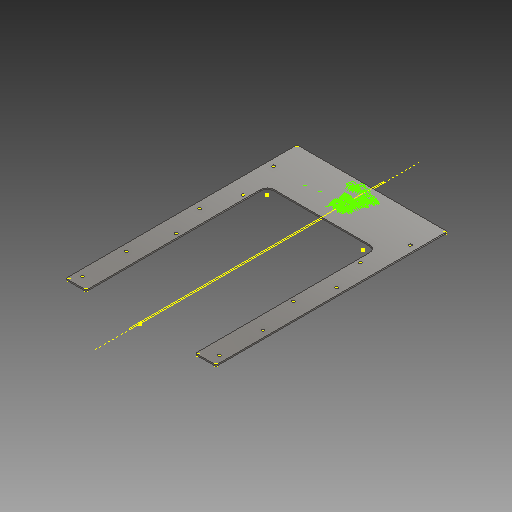
# Autodesk Inventor part: Front
Saved by Autodesk Inventor 2018 (Build 220112000, 112)
## iProperties
Created: 2017-10-08
Part Number: Front
Material: Edelstahl
Document SubType Name: Blech
Designer: jro
Density: 8 g/cm^3
Sheet Metal Rule: Standard_mm
Appearance: Halbpoliert
Mass: 436.49 g
Surface Area: 580.02 cm^2
Volume: 54.5612 cm^3
Flat Pattern Width: 22.4 cm
Flat Pattern Length: 34.5 cm
Flat Pattern Area: 772.799 cm^2
Sheet Metal Width: 224,000 mm
Sheet Metal Length: 345,000 mm
Sheet Metal Area: 77279,943 mm^2
Author: jro
Autodesk Inventor part; units mm, degrees
(part 1 of 2)
ref_plane "YZ Plane" through (0, 0, 0) normal (1, 0, 0) x (0, 1, 0)
ref_plane "XZ Plane" through (0, 0, 0) normal (0, 1, 0) x (-1, 0, 0)
ref_plane "XY Plane" through (0, 0, 0) normal (0, 0, 1) x (1, 0, 0)
sketch "Skizze1" plane through (0, 0, 0) normal (0, 0, 1) x (1, 0, 0)
  line L0 (106.9629, 2) -> (-106.9629, 2)
  line L1 (0, -19.6018) -> (0, 5.6106)
  line L2 (0, 2) -> (81.5, 2)
  line L3 (0, 2) -> (-81.5, 2)
  line L4 (-81.5, 2) -> (-81.5, 262)
  line L5 (81.5, 2) -> (81.5, 262)
  line L6 (71.5, 272) -> (-71.5, 272)
  arc A0 (81.5, 262) -> (71.5, 272) centre (71.5, 262) ccw
  arc A1 (-71.5, 272) -> (-81.5, 262) centre (-71.5, 262) ccw
  line L7 (-81.5, 2) -> (-106.9629, 2)
  line L8 (-106.9629, 2) -> (-106.9629, 347)
  line L9 (81.5, 2) -> (106.9629, 2)
  line L10 (106.9629, 2) -> (106.9629, 347)
  line L11 (106.9629, 347) -> (-106.9629, 347)
  point P0 (0, 0)
  point P1 (-81.5, 272)
  point P2 (81.5, 272)
  point P3 (-106.9629, 347)
  dimension "d7" = 0
  dimension "d0" = 81.5
  dimension "d1" = 81.5
  dimension "PortalHoehe" = 270
  dimension "d3" = 270
  dimension "d4" = 10
  dimension "GesammtHoehe" = 345
  dimension "d6" = 345
  measures "d0" distance of L2.start L2.end
  measures "d1" distance of L2.start L3.end
  measures "PortalHoehe" distance of L3.end point (-81.5, 272)
  measures "d3" distance of L2.end point (81.5, 272)
  measures "d4" radius of A0
  measures "GesammtHoehe" distance of L0.end point (-106.963, 347)
  measures "d6" distance of L0.start point (106.963, 347)
extrude "Grobblech1" add sketch "Skizze1" along normal blind 2 contours L0 L5 A0 L6 A1 L4 L8 L11 L10
fillet "Rundung1" radius 2 2 edges at (-81.5, 2, 1) (81.5, 2, 1)
sketch "Skizze3" plane through (0, 0, 0) normal (0, 0, -1) x (-1, 0, 0)
  arc A0 (-83.5, 2) -> (-81.5, 4) centre (-83.5, 4) ccw projected
  line L0 (-81.5, 262) -> (-81.5, 4) projected
  arc A1 (-71.5, 272) -> (-81.5, 262) centre (-71.5, 262) ccw projected
  line L1 (71.5, 272) -> (-71.5, 272) projected
  arc A2 (81.5, 262) -> (71.5, 272) centre (71.5, 262) ccw projected
  line L2 (81.5, 4) -> (81.5, 262) projected
  arc A3 (81.5, 4) -> (83.5, 2) centre (83.5, 4) ccw projected
  line L3 (106.9629, 2) -> (83.5, 2) projected
  line L4 (106.9629, 347) -> (106.9629, 2) projected
  line L5 (-106.9629, 347) -> (106.9629, 347) projected
  line L6 (-106.9629, 2) -> (-106.9629, 347) projected
  line L7 (-83.5, 2) -> (-106.9629, 2) projected
  circle A4 centre (-87.5, 142) radius 2.15
  circle A5 centre (87.5, 142) radius 2.15
  circle A6 centre (-87.5, 242) radius 2.15
  circle A7 centre (87.5, 242) radius 2.15
  point P0 (0, 0)
  dimension "Durchmesser" = 4.3
  dimension "d23" = 140
  dimension "d24" = 6
  dimension "d25" = 4.3
  dimension "d26" = 6
  dimension "d27" = 140
  dimension "d30" = 4.3
  dimension "d31" = 4.3
  dimension "d32" = 6
  dimension "d33" = 6
  dimension "d34" = 100
  dimension "d35" = 100
  constraints: 4 centre point
  measures "Durchmesser" diameter of A4
  measures "d23" distance from line of L7 A4.centre
  measures "d24" distance from line of L0 A4.centre
  measures "d25" diameter of A5
  measures "d26" distance from line of L2 A5.centre
  measures "d27" distance from line of L3 A5.centre
  measures "d30" diameter of A6
  measures "d31" diameter of A7
  measures "d32" distance from line of L0 A6.centre
  measures "d33" distance from line of L2 A7.centre
  measures "d34" distance of A5.centre A7.centre
  measures "d35" distance of A4.centre A6.centre
extrude "Extrusion3" cut sketch "Skizze3" against normal through all contours A4 | A5 | A6 | A7
ref_plane "Arbeitsebene1" through (0, 2, 0) normal (-1, 0, 0) x (0, 0, 1)
sketch "Skizze4" plane through (0, 0, 0) normal (0, 0, -1) x (-1, 0, 0)
  line L0 (-106.9629, 2) -> (-106.9629, 347) projected
  line L1 (-111.9999, 2) -> (-111.9999, 339.9629)
  line L2 (106.9629, 347) -> (106.9629, 2) projected
  line L3 (111.9999, 339.9629) -> (111.9999, 2)
  line L4 (-106.9629, 2) -> (-83.5, 2) projected
  line L5 (-106.9629, 2) -> (-111.9999, 2)
  line L6 (-111.9999, 2) -> (-111.9999, 347)
  line L7 (-111.9999, 347) -> (-106.9629, 347)
  line L8 (-106.9629, 347) -> (-106.9629, 2)
  line L9 (106.9629, 2) -> (106.9629, 347) projected
  line L10 (106.9629, 2) -> (111.9999, 2)
  line L11 (111.9999, 2) -> (111.9999, 347)
  line L12 (111.9999, 347) -> (106.9629, 347)
  line L13 (106.9629, 347) -> (106.9629, 2)
  point P0 (0, 0)
  dimension "d38" = 223.9998
  dimension "d39" = 345
  constraints: 20 end point, 4 parallel, 2 horizontal, 2 perpendicular, 2 point on line, 2 vertical, 4 other
  measures "d38" distance between parallel lines of L3 L6
  measures "d39" distance between parallel lines of L12 L4
extrude "Extrusion4" add sketch "Skizze4" against normal up to surface (2 mm away)
fillet "Rundung2" radius 2 4 edges at (111.9999, 2, 1) (111.9999, 347, 1) (-111.9999, 347, 1) (-111.9999, 2, 1)
sketch "Skizze6" plane through (0, 0, 0) normal (0, 0, -1) x (-1, 0, 0)
  circle A0 centre (-101.9999, 302) radius 2.15
  circle A1 centre (-101.9999, 192) radius 2.15
  circle A2 centre (-101.9999, 82) radius 2.15
  circle A3 centre (101.9999, 82) radius 2.15
  circle A4 centre (101.9999, 192) radius 2.15
  circle A5 centre (101.9999, 302) radius 2.15
  point P0 (0, 0)
  constraints: 6 centre point, 12 other
extrude "Extrusion5" cut sketch "Skizze6" against normal through all
sketch "Skizze7" plane through (0, 0, 0) normal (0, 0, -1) x (-1, 0, 0)
  circle A0 centre (101.9999, 82) radius 1.9
  line L0 (111.9999, 4) -> (111.9999, 345) projected
  circle A1 centre (101.9999, 17) radius 2.15
  circle A2 centre (101.9999, 82) radius 2.15 projected
  line L1 (109.9999, 2) -> (83.5, 2) projected
  line L2 (0, -69.4) -> (0, 416.4) construction
  circle A3 centre (-101.9999, 17) radius 2.15
  point P0 (0, 0)
  dimension "d45" = 10
  dimension "d46" = 4.3
  dimension "d47" = 4.3
  dimension "d48" = 10
  dimension "d49" = 15
  constraints: 3 centre point, 1 symmetric about line, 3 other
  measures "d45" distance from line of L0 A0.centre
  measures "d46" diameter of A1
  measures "d47" diameter of A2
  measures "d48" distance from line of L0 A1.centre
  measures "d49" distance from line of L1 A1.centre
extrude "Extrusion6" cut sketch "Skizze7" against normal through all contours A1 | A3
sketch "Skizze8" plane through (0, 0, 0) normal (0, 0, -1) x (-1, 0, 0)
  line L0 (96.9499, 289) -> (-96.9499, 289) construction
  line L1 (-110.0001, 345) -> (109.9999, 345) construction
  circle A0 centre (101.9999, 17) radius 2.15 construction
  circle A1 centre (-101.9999, 17) radius 2.15 construction
  circle A2 centre (101.9999, 192) radius 2.15 construction
  circle A3 centre (-101.9999, 82) radius 2.15 construction
  circle A4 centre (-101.9999, 302) radius 2.15 construction
  circle A5 centre (-101.9999, 192) radius 2.15 construction
  circle A6 centre (101.9999, 82) radius 2.15 construction
  circle A7 centre (101.9999, 302) radius 2.15 construction
  circle A8 centre (-87.5, 242) radius 2.15 construction
  circle A9 centre (-87.5, 142) radius 2.15 construction
  circle A10 centre (87.5, 142) radius 2.15 construction
  circle A11 centre (87.5, 242) radius 2.15 construction
  arc A12 (109.9999, 2) -> (111.9999, 4) centre (109.9999, 4) ccw construction
  line L2 (111.9999, 4) -> (111.9999, 345) construction
  arc A13 (111.9999, 345) -> (109.9999, 347) centre (109.9999, 345) ccw construction
  line L3 (-109.9999, 347) -> (109.9999, 347) construction
  arc A14 (-109.9999, 347) -> (-111.9999, 345) centre (-109.9999, 345) ccw construction
  line L4 (-111.9999, 4) -> (-111.9999, 345) construction
  arc A15 (-111.9999, 4) -> (-109.9999, 2) centre (-109.9999, 4) ccw construction
  line L5 (-83.5, 2) -> (-109.9999, 2) construction
  arc A16 (-83.5, 2) -> (-81.5, 4) centre (-83.5, 4) ccw construction
  line L6 (-81.5, 262) -> (-81.5, 4) construction
  arc A17 (-71.5, 272) -> (-81.5, 262) centre (-71.5, 262) ccw construction
  line L7 (71.5, 272) -> (-71.5, 272) construction
  arc A18 (81.5, 262) -> (71.5, 272) centre (71.5, 262) ccw construction
  line L8 (81.5, 4) -> (81.5, 262) construction
  arc A19 (81.5, 4) -> (83.5, 2) centre (83.5, 4) ccw construction
  line L9 (109.9999, 2) -> (83.5, 2) construction
  line L10 (0, -69.4828) -> (0, 416.8971) construction
  line L11 (-21.9888, 341.1437) -> (20.4434, 341.3541) construction
  line L12 (20.4434, 341.3541) -> (20.6916, 291.2842) construction
  line L13 (20.6916, 291.2842) -> (-21.7405, 291.0738) construction
  line L14 (-21.7405, 291.0738) -> (-21.9888, 341.1437) construction
  arc A20 (19.3496, 319.0778) -> (1.9676, 319.3607) centre (10.1704, 289.2139) ccw
  line L15 (1.9676, 319.3607) -> (1.9819, 317.5866)
  line L16 (1.9818, 317.6019) -> (3.6198, 317.3142)
  line L17 (19.3753, 319.1605) -> (18.5828, 316.6107)
  line L18 (18.5828, 316.6107) -> (13.2837, 316.6107)
  arc A21 (13.2837, 316.6107) -> (9.6724, 303.1904) centre (33.9159, 303.8627) ccw
  line L19 (5.4946, 316.1827) -> (4.9509, 316.1827) construction
  line L20 (4.9509, 316.1827) -> (4.4408, 315.289) construction
  line L21 (4.4408, 315.289) -> (3.9664, 313.7628) construction
  line L22 (3.9664, 313.7628) -> (3.5554, 311.6427) construction
  line L23 (3.5554, 311.6427) -> (4.1924, 310.7813) construction
  line L24 (4.1924, 310.7813) -> (5.1161, 310.7813) construction
  line L25 (5.1161, 310.7813) -> (5.5823, 312.2813) construction
  line L26 (5.5823, 312.2813) -> (5.9651, 314.2558) construction
  line L27 (5.9651, 314.2558) -> (6.564, 316.1827) construction
  line L28 (6.564, 316.1827) -> (5.4946, 316.1827) construction
  spline S0 degree 4 poles (5.4946, 316.1827) (4.9509, 316.1827) (4.4408, 315.289) (3.9664, 313.7628) (3.5554, 311.6427) (4.1924, 310.7813) (5.1161, 310.7813) (5.5823, 312.2813) (5.9651, 314.2558) (6.564, 316.1827) (5.4946, 316.1827) knots 1 1 1 1 1 2 3 4 5 6 7 8 8 8 8 8
  spline S1 degree 5 poles (7.5288, 316.1409) (7.3345, 315.9694) (7.2132, 315.5291) (7.665, 314.4803) (6.9392, 313.8958) (7.7886, 312.5748) (6.3912, 310.6819) (8.3951, 311.1239) (9.3384, 310.9161) (10.2863, 311.0182) (10.4883, 312.3413) (10.6389, 313.395) (10.6496, 314.2478) (10.8277, 315.0592) (11.3773, 316.4136) (10.0533, 316.3479) (9.1249, 316.562) (9.063, 316.3507) (8.124, 316.4223) (7.6967, 316.289) (7.5288, 316.1409) knots 0 0 0 0 0 0 0.081449 0.137013 0.205561 0.274127 0.339831 0.403574 0.4666 0.528081 0.588668 0.650647 0.711979 0.770552 0.826478 0.883954 0.929653 1 1 1 1 1 1
  spline S2 degree 5 poles (7.4683, 304.5511) (7.0363, 304.6451) (6.3044, 304.7173) (5.2307, 304.585) (3.7066, 303.5974) (2.4753, 302.9388) (1.1128, 300.0658) (1.1314, 298.3056) (0.4485, 290.255) (10.3579, 292.8549) (10.1936, 296.6226) (11.3006, 298.5778) (10.2295, 301.9983) (9.7797, 303.5426) (8.7017, 304.1824) (7.9281, 304.4511) (7.4683, 304.5511) knots 0 0 0 0 0 0 0.080624 0.134909 0.206036 0.287421 0.381058 0.480825 0.581812 0.683264 0.774591 0.853641 0.914178 1 1 1 1 1 1
  line L29 (10.814, 298.6728) -> (13.0929, 298.6728)
  line L30 (13.0867, 298.6728) -> (13.4054, 296.4373)
  line L31 (13.4054, 296.4373) -> (10.2791, 295.9217)
  line L32 (-4.3084, 300.6806) -> (-4.9654, 298.991) construction
  line L33 (-4.9654, 298.991) -> (-4.6396, 297.5577) construction
  line L34 (-4.6396, 297.5577) -> (-4.3881, 295.7933) construction
  line L35 (-4.3881, 295.7933) -> (-3.3769, 293.8404) construction
  line L36 (-3.3769, 293.8404) -> (-1.555, 292.8006) construction
  line L37 (-1.555, 292.8006) -> (-0.3692, 293.6773) construction
  line L38 (-0.3692, 293.6773) -> (0.3778, 294.755) construction
  line L39 (0.3778, 294.755) -> (1.1836, 295.7372) construction
  spline S3 degree 4 poles (0.493, 299.6585) (-0.5404, 300.713) (-2.403, 301.4871) (-4.3084, 300.6806) (-4.9654, 298.991) (-4.6396, 297.5577) (-4.3881, 295.7933) (-3.3769, 293.8404) (-1.555, 292.8006) (-0.3692, 293.6773) (0.3778, 294.755) (1.1836, 295.7372) knots 1.100161 1.100161 1.100161 1.100161 1.100161 2 3 4 5 6 7 8 9 9 9 9 9
  line L40 (-2.1784, 307.6656) -> (-3.6337, 307.9477) construction
  line L41 (-3.6337, 307.9477) -> (-4.6548, 308.5679) construction
  line L42 (-9.2107, 309.4764) -> (-10.879, 308.8022) construction
  line L43 (-10.879, 308.8022) -> (-12.9465, 307.6935) construction
  line L44 (-12.9465, 307.6935) -> (-14.3475, 306.7475) construction
  line L45 (-14.3475, 306.7475) -> (-15.1878, 306.079) construction
  line L46 (-15.1878, 306.079) -> (-14.4016, 304.1368) construction
  line L47 (-14.4016, 304.1368) -> (-13.5488, 302.0298) construction
  line L48 (-13.5488, 302.0298) -> (-12.4435, 299.8953) construction
  line L49 (-10.0091, 293.0182) -> (-8.5191, 292.1678) construction
  line L50 (-8.5191, 292.1678) -> (-6.6934, 292.2248) construction
  line L51 (-6.6934, 292.2248) -> (-5.8633, 293.9743) construction
  line L52 (-5.8633, 293.9743) -> (-5.3186, 295.7267) construction
  line L53 (-5.3186, 295.7267) -> (-5.3186, 297.1959) construction
  line L54 (-5.3186, 297.1959) -> (-6.038, 298.9733) construction
  line L55 (-6.038, 298.9733) -> (-7.8901, 300.0304) construction
  line L56 (-7.8901, 300.0304) -> (-10.1449, 299.5179) construction
  line L57 (-10.1449, 299.5179) -> (-11.0423, 296.4952) construction
  line L58 (-11.0423, 296.4952) -> (-12.3256, 296.6461) construction
  line L59 (-12.3256, 296.6461) -> (-13.9407, 295.8151) construction
  line L60 (-13.9407, 295.8151) -> (-13.9407, 295.0935) construction
  line L61 (-13.9407, 295.0935) -> (-13.2651, 293.4244) construction
  line L62 (-13.2651, 293.4244) -> (-12.4049, 294.0604) construction
  line L63 (-12.4049, 294.0604) -> (-11.3216, 294.4296) construction
  line L64 (-11.3216, 294.4296) -> (-10.9103, 294.8751) construction
  spline S4 degree 4 poles (-11.0423, 296.4952) (-12.3256, 296.6461) (-13.9407, 295.8151) (-13.9407, 295.0935) (-13.2651, 293.4244) (-12.4049, 294.0604) (-11.3216, 294.4296) (-10.9103, 294.8751) knots 1 1 1 1 1 2 3 4 5 5 5 5 5
  line L65 (-7.4842, 296.3019) -> (-7.166, 296.4307) construction
  line L66 (-7.166, 296.4307) -> (-7.6609, 297.6535) construction
  line L67 (-7.6609, 297.6535) -> (-8.6673, 297.6535) construction
  line L68 (-8.6673, 297.6535) -> (-9.1528, 296.8029) construction
  line L69 (-9.1528, 296.8029) -> (-9.1528, 295.6336) construction
  line L70 (-9.1528, 295.6336) -> (-8.3414, 295.1705) construction
  line L71 (-8.3414, 295.1705) -> (-7.4984, 295.5117) construction
  line L72 (-7.4984, 295.5117) -> (-6.8817, 295.9676) construction
  line L73 (-6.8817, 295.9676) -> (-6.0959, 296.5486) construction
  line L74 (-6.0959, 296.5486) -> (-5.6756, 296.7442) construction
  line L75 (-5.6756, 296.7442) -> (-3.894, 296.9982) construction
  line L76 (-3.894, 296.9982) -> (-2.9759, 297.3698) construction
  line L77 (-2.9759, 297.3698) -> (-2.0239, 296.3946) construction
  line L78 (-2.0239, 296.3946) -> (-1.188, 297.3411) construction
  line L79 (-1.188, 297.3411) -> (-1.188, 298.4259) construction
  line L80 (-1.188, 298.4259) -> (-2.1576, 298.0321) construction
  line L81 (-2.1576, 298.0321) -> (-2.3947, 298.6818) construction
  line L82 (-2.3947, 298.6818) -> (-3.5332, 297.84) construction
  line L83 (-3.5332, 297.84) -> (-4.5133, 297.5044) construction
  line L84 (-4.5133, 297.5044) -> (-5.7568, 297.0011) construction
  line L85 (-5.7568, 297.0011) -> (-6.933, 296.5251) construction
  line L86 (-6.933, 296.5251) -> (-7.4842, 296.3019) construction
  spline S5 degree 4 poles (-7.4842, 296.3019) (-7.166, 296.4307) (-7.6609, 297.6535) (-8.6673, 297.6535) (-9.1528, 296.8029) (-9.1528, 295.6336) (-8.3414, 295.1705) (-7.4984, 295.5117) (-6.8817, 295.9676) (-6.0959, 296.5486) (-5.6756, 296.7442) (-3.894, 296.9982) (-2.9759, 297.3698) (-2.0239, 296.3946) (-1.188, 297.3411) (-1.188, 298.4259) (-2.1576, 298.0321) (-2.3947, 298.6818) (-3.5332, 297.84) (-4.5133, 297.5044) (-5.7568, 297.0011) (-6.933, 296.5251) (-7.4842, 296.3019) knots 1 1 1 1 1 2 3 4 5 6 7 8 9 10 11 12 13 14 15 16 17 18 19 20 20 20 20 20
  line L87 (5.6915, 299.3238) -> (5.1012, 299.0055) construction
  line L88 (4.957, 297.7916) -> (5.598, 297.4097) construction
  line L89 (-0.0145, 312.4222) -> (-0.2397, 314.0262) construction
  line L90 (-0.2397, 314.0262) -> (-1.4991, 314.9371) construction
  line L91 (-1.4991, 314.9371) -> (-2.639, 314.4757) construction
  line L92 (-2.639, 314.4757) -> (-3.7779, 313.6336) construction
  spline S6 degree 4 poles (1.3739, 310.428) (0.994, 310.6163) (0.5638, 311.5994) (-0.0145, 312.4222) (-0.2397, 314.0262) (-1.4991, 314.9371) (-2.639, 314.4757) (-3.7779, 313.6336) (-3.873, 312.6815) (-3.9514, 312.0076) (-4.0017, 311.7338) knots 1.199698 1.199698 1.199698 1.199698 1.199698 2 3 4 5 6 7 7.655091 7.655091 7.655091 7.655091 7.655091
  line L93 (-7.8752, 309.8047) -> (-7.6878, 310.8485) construction
  line L94 (-7.6878, 310.8485) -> (-9.0138, 310.9359) construction
  line L95 (-9.0138, 310.9359) -> (-9.7726, 310.8558) construction
  line L96 (-9.7726, 310.8558) -> (-11.8503, 310.2971) construction
  line L97 (-11.8503, 310.2971) -> (-13.2342, 309.5891) construction
  line L98 (-13.2342, 309.5891) -> (-14.6404, 308.7695) construction
  line L99 (-14.6404, 308.7695) -> (-13.6109, 307.2449) construction
  spline S7 degree 4 poles (-7.8752, 309.8047) (-7.6878, 310.8485) (-9.0138, 310.9359) (-9.7726, 310.8558) (-11.8503, 310.2971) (-13.2342, 309.5891) (-14.6404, 308.7695) (-13.6109, 307.2449) knots 1 1 1 1 1 2 3 4 5 5 5 5 5
  line L100 (-8.5107, 310.8588) -> (-8.2741, 311.1796) construction
  line L101 (-8.2741, 311.1796) -> (-8.5243, 312.9345) construction
  line L102 (-8.5243, 312.9345) -> (-8.2592, 314.6576) construction
  line L103 (-8.2592, 314.6576) -> (-8.4691, 316.7623) construction
  line L104 (-8.4691, 316.7623) -> (-7.9694, 317.9259) construction
  line L105 (-7.9694, 317.9259) -> (-6.5636, 318.2188) construction
  line L106 (-6.5636, 318.2188) -> (-6.6312, 319.0827) construction
  line L107 (-6.6312, 319.0827) -> (-6.497, 319.8488) construction
  line L108 (-6.497, 319.8488) -> (-6.7278, 320.4188) construction
  line L109 (-6.7278, 320.4188) -> (-8.5451, 320.4188) construction
  line L110 (-8.5451, 320.4188) -> (-11.067, 320.2724) construction
  line L111 (-11.067, 320.2724) -> (-13.375, 320.0134) construction
  line L112 (-13.375, 320.0134) -> (-15.5889, 319.2126) construction
  line L113 (-15.5889, 319.2126) -> (-17.6144, 317.6111) construction
  line L114 (-17.6144, 317.6111) -> (-20.4642, 316.2922) construction
  line L115 (-20.4642, 316.2922) -> (-18.2738, 314.3845) construction
  line L116 (-18.2738, 314.3845) -> (-17.2636, 315.0661) construction
  line L117 (-17.2636, 315.0661) -> (-16.3096, 313.7759) construction
  line L118 (-16.3096, 313.7759) -> (-15.3841, 312.5242) construction
  line L119 (-15.3841, 312.5242) -> (-14.1615, 310.8659) construction
  line L120 (-14.1615, 310.8659) -> (-13.6935, 309.7353) construction
  line L121 (-13.6935, 309.7353) -> (-14.099, 308.5303) construction
  spline S8 degree 4 poles (-8.5107, 310.8588) (-8.2741, 311.1796) (-8.5243, 312.9345) (-8.2592, 314.6576) (-8.4691, 316.7623) (-7.9694, 317.9259) (-6.5636, 318.2188) (-6.6312, 319.0827) (-6.497, 319.8488) (-6.7278, 320.4188) (-8.5451, 320.4188) (-11.067, 320.2724) (-13.375, 320.0134) (-15.5889, 319.2126) (-17.6144, 317.6111) (-20.4642, 316.2922) (-18.2738, 314.3845) (-17.2636, 315.0661) (-16.3096, 313.7759) (-15.3841, 312.5242) (-14.1615, 310.8659) (-13.6935, 309.7353) (-14.099, 308.5303) knots 1 1 1 1 1 2 3 4 5 6 7 8 9 10 11 12 13 14 15 16 17 18 19 20 20 20 20 20
  line L122 (-17.7343, 314.7458) -> (-14.8581, 317.8309) construction
  line L123 (-14.8581, 317.8309) -> (-10.7977, 319.2486) construction
  line L124 (-10.7977, 319.2486) -> (-7.2665, 318.0724) construction
  spline S9 degree 3 poles (-17.7343, 314.7458) (-14.8581, 317.8309) (-10.7977, 319.2486) (-7.2665, 318.0724) knots 1 1 1 1 2 2 2 2
  line L125 (-17.8071, 327.5617) -> (-18.42, 329.0758) construction
  line L126 (-18.42, 329.0758) -> (-16.8783, 329.6998) construction
  line L127 (-16.8783, 329.6998) -> (-16.8357, 331.7501) construction
  line L128 (-16.8357, 331.7501) -> (-11.7164, 333.2196) construction
  line L129 (-11.7164, 333.2196) -> (-11.0291, 330.1148) construction
  line L130 (-11.0291, 330.1148) -> (-7.3761, 331.7428) construction
  line L131 (-7.3761, 331.7428) -> (-7.3761, 330.666) construction
  line L132 (-7.3761, 330.666) -> (-5.1723, 329.4082) construction
  line L133 (-5.1723, 329.4082) -> (-6.4181, 328.9039) construction
  line L134 (-6.4181, 328.9039) -> (-6.0969, 326.6509) construction
  line L135 (-6.0969, 326.6509) -> (-6.8104, 325.8961) construction
  line L136 (-6.8104, 325.8961) -> (-5.4239, 324.4724) construction
  line L137 (-5.4239, 324.4724) -> (-7.0299, 323.2849) construction
  line L138 (-7.0299, 323.2849) -> (-8.7981, 322.4236) construction
  line L139 (-8.7981, 322.4236) -> (-9.7338, 324.2807) construction
  line L140 (-9.7338, 324.2807) -> (-11.6168, 324.0985) construction
  line L141 (-11.6168, 324.0985) -> (-11.4677, 322.5227) construction
  line L142 (-11.4677, 322.5227) -> (-13.2569, 321.867) construction
  line L143 (-13.2569, 321.867) -> (-14.9162, 321.5934) construction
  line L144 (-14.9162, 321.5934) -> (-17.4443, 323.0362) construction
  line L145 (-17.4443, 323.0362) -> (-19.4217, 322.2358) construction
  line L146 (-19.4217, 322.2358) -> (-21.0945, 323.1905) construction
  line L147 (-21.0945, 323.1905) -> (-21.0945, 324.3118) construction
  line L148 (-21.0945, 324.3118) -> (-21.0945, 326.1023) construction
  line L149 (-21.0945, 326.1023) -> (-20.0222, 326.1023) construction
  line L150 (-20.0222, 326.1023) -> (-19.7279, 327.7834) construction
  line L151 (-19.7279, 327.7834) -> (-17.8071, 327.5617) construction
  spline S10 degree 4 poles (-17.8071, 327.5617) (-18.42, 329.0758) (-16.8783, 329.6998) (-16.8357, 331.7501) (-11.7164, 333.2196) (-11.0291, 330.1148) (-7.3761, 331.7428) (-7.3761, 330.666) (-5.1723, 329.4082) (-6.4181, 328.9039) (-6.0969, 326.6509) (-6.8104, 325.8961) (-5.4239, 324.4724) (-7.0299, 323.2849) (-8.7981, 322.4236) (-9.7338, 324.2807) (-11.6168, 324.0985) (-11.4677, 322.5227) (-13.2569, 321.867) (-14.9162, 321.5934) (-17.4443, 323.0362) (-19.4217, 322.2358) (-21.0945, 323.1905) (-21.0945, 324.3118) (-21.0945, 326.1023) (-20.0222, 326.1023) (-19.7279, 327.7834) (-17.8071, 327.5617) knots 1 1 1 1 1 2 3 4 5 6 7 8 9 10 11 12 13 14 15 16 17 18 19 20 21 22 23 24 25 25 25 25 25
  line L152 (0.0671, 337.5212) -> (6.9996, 338.5829) construction
  line L153 (6.9996, 338.5829) -> (9.7158, 340.5912) construction
  line L154 (9.7158, 340.5912) -> (7.9669, 338.8128) construction
  line L155 (7.9669, 338.8128) -> (11.545, 336.8612) construction
  line L156 (11.545, 336.8612) -> (11.3946, 334.1807) construction
  line L157 (11.3946, 334.1807) -> (9.1146, 332.9208) construction
  line L158 (9.1146, 332.9208) -> (11.4176, 331.6064) construction
  line L159 (11.4176, 331.6064) -> (13.3497, 333.0349) construction
  line L160 (13.3497, 333.0349) -> (14.4768, 330.2503) construction
  line L161 (14.4768, 330.2503) -> (12.9563, 334.0068) construction
  line L162 (12.9563, 334.0068) -> (19.9715, 336.8462) construction
  line L163 (19.9715, 336.8462) -> (21.2069, 333.7939) construction
  line L164 (21.2069, 333.7939) -> (18.3758, 332.6479) construction
  line L165 (18.3758, 332.6479) -> (16.7995, 329.5516) construction
  line L166 (16.7995, 329.5516) -> (13.0943, 328.276) construction
  line L167 (13.0943, 328.276) -> (14.5593, 331.5513) construction
  line L168 (14.5593, 331.5513) -> (11.8877, 330.47) construction
  line L169 (11.8877, 330.47) -> (11.8877, 329.8437) construction
  line L170 (11.8877, 329.8437) -> (9.9637, 329.065) construction
  line L171 (9.9637, 329.065) -> (9.2971, 330.712) construction
  line L172 (9.2971, 330.712) -> (9.2971, 331.4816) construction
  line L173 (9.2971, 331.4816) -> (7.5185, 330.7618) construction
  line L174 (7.5185, 330.7618) -> (6.0484, 328.6405) construction
  line L175 (6.0484, 328.6405) -> (5.4168, 331.6903) construction
  line L176 (5.4168, 331.6903) -> (3.9436, 331.094) construction
  line L177 (3.9436, 331.094) -> (2.2825, 332.3457) construction
  line L178 (2.2825, 332.3457) -> (0.919, 330.392) construction
  line L179 (0.919, 330.392) -> (-1.6048, 331.556) construction
  line L180 (-1.6048, 331.556) -> (0.5211, 333.5605) construction
  line L181 (0.5211, 333.5605) -> (-2.1515, 334.9575) construction
  line L182 (-2.1515, 334.9575) -> (0.1798, 337.5384) construction
  line L183 (0.1798, 337.5384) -> (2.7458, 337.9314) construction
  spline S11 degree 4 poles (0.0671, 337.5212) (6.9996, 338.5829) (9.7158, 340.5912) (7.9669, 338.8128) (11.545, 336.8612) (11.3946, 334.1807) (9.1146, 332.9208) (11.4176, 331.6064) (13.3497, 333.0349) (14.4768, 330.2503) (12.9563, 334.0068) (19.9715, 336.8462) (21.2069, 333.7939) (18.3758, 332.6479) (16.7995, 329.5516) (13.0943, 328.276) (14.5593, 331.5513) (11.8877, 330.47) (11.8877, 329.8437) (9.9637, 329.065) (9.2971, 330.712) (9.2971, 331.4816) (7.5185, 330.7618) (6.0484, 328.6405) (5.4168, 331.6903) (3.9436, 331.094) (2.2825, 332.3457) (0.919, 330.392) (-1.6048, 331.556) (0.5211, 333.5605) (-2.1515, 334.9575) (0.1798, 337.5384) (2.7458, 337.9314) knots 1 1 1 1 1 2 3 4 5 6 7 8 9 10 11 12 13 14 15 16 17 18 19 20 21 22 23 24 25 26 27 28 29 30 30 30 30 30
  line L184 (-20.2856, 326.2295) -> (-21.0128, 328.0263) construction
  line L185 (-21.0128, 328.0263) -> (-16.8783, 329.6998) construction
  line L186 (-16.8783, 329.6998) -> (-16.8357, 331.7501) construction
  line L187 (-16.8357, 331.7501) -> (-11.7164, 333.2196) construction
  line L188 (-11.7164, 333.2196) -> (-11.0291, 330.1148) construction
  line L189 (-11.0291, 330.1148) -> (-7.3761, 331.7428) construction
  line L190 (-7.3761, 331.7428) -> (-7.3761, 330.666) construction
  line L191 (-7.3761, 330.666) -> (-5.1723, 329.4082) construction
  line L192 (-5.1723, 329.4082) -> (-6.4181, 328.9039) construction
  line L193 (-6.4181, 328.9039) -> (-6.0969, 326.6509) construction
  line L194 (-6.0969, 326.6509) -> (-6.8104, 325.8961) construction
  line L195 (-6.8104, 325.8961) -> (-5.4239, 324.4724) construction
  line L196 (-5.4239, 324.4724) -> (-7.0299, 323.2849) construction
  line L197 (-7.0299, 323.2849) -> (-8.7981, 322.4236) construction
  line L198 (-8.7981, 322.4236) -> (-9.7338, 324.2807) construction
  line L199 (-9.7338, 324.2807) -> (-11.6168, 324.0985) construction
  line L200 (-11.6168, 324.0985) -> (-11.4677, 322.5227) construction
  line L201 (-11.4677, 322.5227) -> (-13.2569, 321.867) construction
  line L202 (-13.2569, 321.867) -> (-14.9162, 321.5934) construction
  line L203 (-14.9162, 321.5934) -> (-17.4443, 323.0362) construction
  line L204 (-17.4443, 323.0362) -> (-19.4217, 322.2358) construction
  line L205 (-19.4217, 322.2358) -> (-21.0945, 323.1905) construction
  line L206 (-21.0945, 323.1905) -> (-21.0945, 324.3118) construction
  line L207 (-21.0945, 324.3118) -> (-21.0945, 327.4268) construction
  line L208 (-21.0945, 327.4268) -> (-21.9104, 327.4268) construction
  line L209 (-21.9104, 327.4268) -> (-21.5654, 329.3914) construction
  line L210 (-21.5654, 329.3914) -> (-20.8416, 327.6032) construction
  spline S12 degree 4 poles (-20.2856, 326.2295) (-21.0128, 328.0263) (-16.8783, 329.6998) (-16.8357, 331.7501) (-11.7164, 333.2196) (-11.0291, 330.1148) (-7.3761, 331.7428) (-7.3761, 330.666) (-5.1723, 329.4082) (-6.4181, 328.9039) (-6.0969, 326.6509) (-6.8104, 325.8961) (-5.4239, 324.4724) (-7.0299, 323.2849) (-8.7981, 322.4236) (-9.7338, 324.2807) (-11.6168, 324.0985) (-11.4677, 322.5227) (-13.2569, 321.867) (-14.9162, 321.5934) (-17.4443, 323.0362) (-19.4217, 322.2358) (-21.0945, 323.1905) (-21.0945, 324.3118) (-21.0945, 327.4268) (-21.9104, 327.4268) (-21.5654, 329.3914) (-20.8416, 327.6032) knots 1 1 1 1 1 2 3 4 5 6 7 8 9 10 11 12 13 14 15 16 17 18 19 20 21 22 23 24 25 25 25 25 25
  line L211 (10.6919, 314.2736) -> (11.2088, 314.2736)
  line L212 (11.2088, 314.2736) -> (11.8429, 313.9118)
  line L213 (7.3154, 313.8618) -> (5.9769, 314.1005)
  line L214 (4.1249, 314.1552) -> (2.795, 314.5685)
  line L215 (1.539, 298.168) -> (4.8307, 298.167)
  arc A22 (19.9119, 319.2893) -> (1.5944, 319.6422) centre (10.1704, 289.2139) ccw
  line L216 (1.5944, 319.6422) -> (1.611, 317.5836)
  line L217 (19.9026, 319.2924) -> (18.9247, 316.1464)
  line L218 (18.9247, 316.1464) -> (13.5442, 316.1464)
  arc A23 (13.5442, 316.1464) -> (10.1365, 303.2033) centre (33.9159, 303.8627) ccw
  line L219 (7.2418, 313.4496) -> (5.8989, 313.6891)
  line L220 (4.0158, 313.7994) -> (2.6845, 314.2131)
  line L221 (11.6701, 313.6089) -> (11.1163, 313.9249)
  line L222 (11.1163, 313.9249) -> (10.6919, 313.9249)
  line L223 (10.8144, 299.0286) -> (13.4505, 299.0286)
  line L224 (13.4505, 299.0286) -> (13.8683, 296.0977)
  line L225 (13.8683, 296.0977) -> (10.1037, 295.4768)
  line L226 (1.5824, 298.6833) -> (4.9017, 298.6823)
  spline S13 degree 4 poles (1.2836, 309.9265) (0.5963, 309.3694) (-0.5844, 308.2768) (-2.1784, 307.6656) (-3.6337, 307.9477) (-4.6548, 308.5679) (-5.1837, 309.2009) (-5.4868, 309.4829) (-5.5884, 309.5635) knots 1.158307 1.158307 1.158307 1.158307 1.158307 2 3 4 5 5.494281 5.494281 5.494281 5.494281 5.494281
  line L227 (-4.6548, 308.5679) -> (-5.1837, 309.2009) construction
  line L228 (-5.1837, 309.2009) -> (-5.4868, 309.4829) construction
  line L229 (-5.4868, 309.4829) -> (-5.5884, 309.5635) construction
  line L230 (-8.2859, 309.752) -> (-9.2107, 309.4764) construction
  line L231 (-7.5648, 309.8585) -> (-8.2859, 309.752) construction
  line L232 (-7.297, 309.8999) -> (-7.5648, 309.8585) construction
  spline S14 degree 4 poles (-7.297, 309.8999) (-7.5648, 309.8585) (-8.2859, 309.752) (-9.2107, 309.4764) (-10.879, 308.8022) (-12.9465, 307.6935) (-14.3475, 306.7475) (-15.1878, 306.079) (-14.4016, 304.1368) (-13.5488, 302.0298) (-12.4435, 299.8953) (-11.6313, 298.7436) (-11.3609, 298.0377) (-11.2748, 297.6921) knots 7.026305 7.026305 7.026305 7.026305 7.026305 8 9 10 11 12 13 14 15 16 16.901836 16.901836 16.901836 16.901836 16.901836
  spline S15 degree 4 poles (-10.9103, 294.8751) (-10.8536, 294.6501) (-10.6371, 293.9869) (-10.0091, 293.0182) (-8.5191, 292.1678) (-6.6934, 292.2248) (-5.8633, 293.9743) (-5.3186, 295.7267) (-5.3186, 297.1959) (-6.038, 298.9733) (-7.8901, 300.0304) (-10.1449, 299.5179) (-11.0423, 296.4952) knots 18.506362 18.506362 18.506362 18.506362 18.506362 19 20 21 22 23 24 25 26 27 27 27 27 27
  line L233 (-10.6371, 293.9869) -> (-10.0091, 293.0182) construction
  line L234 (-10.8536, 294.6501) -> (-10.6371, 293.9869) construction
  line L235 (-10.9103, 294.8751) -> (-10.8536, 294.6501) construction
  line L236 (5.6915, 299.3238) -> (5.9021, 298.9333)
  line L237 (5.8251, 297.7909) -> (5.5947, 297.4116)
  spline S16 degree 2 poles (5.6915, 299.3238) (5.1012, 299.0055) (4.9017, 298.6823) knots 0 0 0 1 1 1
  spline S17 degree 2 poles (4.8307, 298.167) (4.957, 297.7916) (5.598, 297.4097) knots 0 0 0 1 1 1
  line L238 (5.1012, 299.0055) -> (4.9017, 298.6823) construction
  line L239 (4.8307, 298.167) -> (4.957, 297.7916) construction
  arc A24 (5.9021, 298.9333) -> (5.8251, 297.7909) centre (5.8395, 298.3637) ccw
  line L240 (-12.4435, 299.8953) -> (-11.6313, 298.7436) construction
  line L241 (-11.6313, 298.7436) -> (-11.3609, 298.0377) construction
  line L242 (-11.3609, 298.0377) -> (-11.2748, 297.6921) construction
  arc A25 (-5.5884, 309.5636) -> (-7.1899, 309.2254) centre (-5.7194, 306.2225) ccw
  arc A26 (-7.2942, 309.8999) -> (-3.9285, 311.8375) centre (-7.628, 314.3716) ccw
  line L243 (-3.7779, 313.6336) -> (-3.873, 312.6815) construction
  line L244 (-3.873, 312.6815) -> (-3.9514, 312.0076) construction
  line L245 (-3.9514, 312.0076) -> (-4.0017, 311.7338) construction
  arc A27 (-5.2661, 309.9694) -> (-3.492, 311.6401) centre (-5.2609, 311.7412) ccw
  line L246 (1.8939, 317.0998) -> (2.9967, 316.9061)
  line L247 (1.611, 317.5836) -> (1.615, 317.0927)
  line L248 (1.615, 317.0927) -> (1.8937, 317.0992)
  line L249 (1.2836, 309.9265) -> (0.5963, 309.3694) construction
  line L250 (0.5963, 309.3694) -> (-0.5844, 308.2768) construction
  line L251 (-0.5844, 308.2768) -> (-2.1784, 307.6656) construction
  line L252 (1.3739, 310.428) -> (0.994, 310.6163) construction
  line L253 (0.994, 310.6163) -> (0.5638, 311.5994) construction
  line L254 (0.5638, 311.5994) -> (-0.0145, 312.4222) construction
  arc A28 (2.9967, 316.9061) -> (1.3739, 310.428) centre (53.9065, 300.7103) ccw
  arc A29 (1.2836, 309.9265) -> (0.701, 295.8845) centre (53.9065, 300.7103) ccw
  arc A30 (3.6198, 317.3142) -> (2.795, 314.5685) centre (53.9065, 300.7103) ccw
  arc A31 (2.6988, 314.2087) -> (1.1836, 295.7372) centre (53.9065, 300.7103) ccw
  line L255 (0.493, 299.6585) -> (-0.5404, 300.713) construction
  line L256 (-0.5404, 300.713) -> (-2.403, 301.4871) construction
  line L257 (-2.403, 301.4871) -> (-4.3084, 300.6806) construction
  arc A32 (0.521, 298.6861) -> (0.1595, 299.3317) centre (-0.1698, 298.7233) ccw
  spline S18 degree 5 poles (-7.8223, 311.1902) (-7.8023, 311.3689) (-7.7974, 311.5491) (-7.7991, 311.7279) (-7.8099, 312.1873) (-7.831, 312.6443) (-7.8391, 312.9239) (-7.8381, 313.4437) (-7.8181, 313.9638) (-7.8082, 314.2046) (-7.7923, 314.6615) (-7.7858, 315.1185) (-7.7851, 315.3344) (-7.7874, 315.7166) (-7.7829, 316.099) (-7.7775, 316.2653) (-7.7603, 316.5345) (-7.7114, 316.7995) (-7.6866, 316.8993) (-7.6279, 317.0666) (-7.5269, 317.2115) (-7.4762, 317.2649) (-7.3406, 317.3795) (-7.1865, 317.4686) (-7.0941, 317.5168) (-6.8755, 317.629) (-6.6638, 317.7532) (-6.5473, 317.8346) (-6.3358, 318.0251) (-6.1833, 318.2655) (-6.1261, 318.3969) (-6.0636, 318.6257) (-6.0356, 318.8607) (-6.0283, 318.9559) (-6.0166, 319.1335) (-6.006, 319.3112) (-6.0005, 319.3936) (-5.9902, 319.5811) (-5.9925, 319.7688) (-6.0005, 319.8739) (-6.0444, 320.1248) (-6.1529, 320.357) (-6.2425, 320.4803) (-6.4674, 320.6905) (-6.7484, 320.8175) (-6.8988, 320.8619) (-7.2309, 320.9314) (-7.5694, 320.9576) (-7.7522, 320.9653) (-8.1566, 320.9725) (-8.5609, 320.9648) (-8.7822, 320.9582) (-9.2485, 320.9402) (-9.7145, 320.9154) (-9.9594, 320.901) (-10.455, 320.8688) (-10.95, 320.8299) (-11.2004, 320.8081) (-11.6997, 320.7596) (-12.1976, 320.6975) (-12.4455, 320.6624) (-12.9423, 320.5809) (-13.4343, 320.4748) (-13.68, 320.4143) (-14.1734, 320.2762) (-14.6562, 320.1047) (-14.8975, 320.009) (-15.3774, 319.7961) (-15.841, 319.5495) (-16.0711, 319.417) (-16.5298, 319.1379) (-16.9796, 318.8449) (-17.2066, 318.6961) (-17.6728, 318.3975) (-18.1433, 318.1052) (-18.3832, 317.9569) (-18.8607, 317.6589) (-19.314, 317.3269) (-19.531, 317.148) (-19.9129, 316.7168) (-20.0783, 316.1616) (-20.0713, 315.8575) (-19.905, 315.3419) (-19.5613, 314.9281) (-19.3777, 314.7611) (-19.0152, 314.4959) (-18.6042, 314.3164) (-18.4124, 314.254) (-18.1156, 314.1949) (-17.8144, 314.1765) (-17.7143, 314.1705) (-17.5483, 314.1706) (-17.3951, 314.107) (-17.345, 314.0692) (-17.1971, 313.9507) (-17.0712, 313.8066) (-16.9882, 313.7099) (-16.8054, 313.4801) (-16.6294, 313.2459) (-16.5313, 313.1129) (-16.317, 312.8234) (-16.1031, 312.5335) (-15.9871, 312.3767) (-15.7352, 312.0339) (-15.4868, 311.6885) (-15.3543, 311.5002) (-15.0945, 311.1209) (-14.8506, 310.7314) (-14.7328, 310.5348) (-14.4961, 310.0729) (-14.4285, 309.5499) (-14.4855, 309.2567) (-14.5482, 308.985) (-14.6413, 308.7128) knots 0 0 0 0 0 0 0.025227 0.025227 0.025227 0.064411 0.064411 0.064411 0.098291 0.098291 0.098291 0.128616 0.128616 0.128616 0.151998 0.151998 0.151998 0.166417 0.166417 0.166417 0.176622 0.176622 0.176622 0.191292 0.191292 0.191292 0.21111 0.21111 0.21111 0.230894 0.230894 0.230894 0.244295 0.244295 0.244295 0.255901 0.255901 0.255901 0.270653 0.270653 0.270653 0.291459 0.291459 0.291459 0.313339 0.313339 0.313339 0.339042 0.339042 0.339042 0.370138 0.370138 0.370138 0.404599 0.404599 0.404599 0.4399 0.4399 0.4399 0.475071 0.475071 0.475071 0.510587 0.510587 0.510587 0.547008 0.547008 0.547008 0.584297 0.584297 0.584297 0.622418 0.622418 0.622418 0.662084 0.662084 0.662084 0.701377 0.701377 0.701377 0.741219 0.741219 0.741219 0.775782 0.775782 0.775782 0.803885 0.803885 0.803885 0.818106 0.818106 0.818106 0.826761 0.826761 0.826761 0.844755 0.844755 0.844755 0.867953 0.867953 0.867953 0.895358 0.895358 0.895358 0.927712 0.927712 0.927712 0.959916 0.959916 0.959916 1 1 1 1 1 1
  spline S19 degree 5 poles (-17.3982, 314.4324) (-16.6085, 315.2796) (-15.7229, 316.0377) (-14.7524, 316.6889) (-12.7483, 317.6866) (-10.5512, 318.0911) (-9.4765, 318.1263) (-8.4137, 317.9702) (-7.4118, 317.6364) knots 0 0 0 0 0 0 0.522987 0.522987 0.522987 1 1 1 1 1 1
  spline S20 degree 5 poles (-7.297, 309.8999) (-7.2733, 310.1341) (-7.2795, 310.3712) (-7.3291, 310.6105) (-7.5358, 311.0041) (-7.8915, 311.2597) (-8.0737, 311.3389) (-8.3893, 311.421) (-8.7146, 311.445) (-8.846, 311.4472) (-9.0851, 311.4433) (-9.3234, 311.4266) (-9.4304, 311.4169) (-9.6418, 311.392) (-9.852, 311.3579) (-9.9557, 311.3388) (-10.17, 311.2957) (-10.3829, 311.246) (-10.4928, 311.2189) (-10.7225, 311.1594) (-10.951, 311.0948) (-11.0702, 311.0597) (-11.3156, 310.9843) (-11.5591, 310.903) (-11.6842, 310.8594) (-11.9393, 310.7666) (-12.1917, 310.6666) (-12.3202, 310.6135) (-12.5841, 310.4997) (-12.8449, 310.3787) (-12.9786, 310.3139) (-13.2716, 310.1693) (-13.5599, 310.0153) (-13.7152, 309.9275) (-14.0774, 309.6912) (-14.3836, 309.384) (-14.5283, 309.1656) (-14.7431, 308.5607) (-14.6258, 307.9135) (-14.4658, 307.5688) (-14.2854, 307.242) (-14.0747, 306.9317) knots 0 0 0 0 0 0 0.105364 0.105364 0.105364 0.191866 0.191866 0.191866 0.250685 0.250685 0.250685 0.298714 0.298714 0.298714 0.345886 0.345886 0.345886 0.396485 0.396485 0.396485 0.452056 0.452056 0.452056 0.511309 0.511309 0.511309 0.573465 0.573465 0.573465 0.639888 0.639888 0.639888 0.719635 0.719635 0.719635 0.832555 0.832555 0.832555 1 1 1 1 1 1
  spline S21 degree 5 poles (0.701, 295.8846) (0.4314, 295.5528) (0.1663, 295.2163) (-0.0976, 294.8837) (-0.4837, 294.3706) (-0.9696, 293.9567) (-1.1429, 293.8359) (-1.5237, 293.678) (-1.9305, 293.7297) (-2.1103, 293.7955) (-2.5012, 293.9963) (-2.8317, 294.2898) (-3.0012, 294.4736) (-3.3144, 294.8807) (-3.5592, 295.3318) (-3.6689, 295.5713) (-3.8515, 296.0477) (-3.985, 296.5403) (-4.0388, 296.7815) (-4.1322, 297.2395) (-4.214, 297.6999) (-4.2506, 297.9172) (-4.312, 298.3248) (-4.3254, 298.7366) (-4.315, 298.9286) (-4.2446, 299.3304) (-4.0701, 299.6996) (-3.948, 299.8793) (-3.6007, 300.2568) (-3.145, 300.5046) (-2.8564, 300.5932) (-1.9951, 300.703) (-1.145, 300.4118) (-0.6681, 300.0931) (-0.2342, 299.735) (0.1595, 299.3317) knots 0 0 0 0 0 0 0.139392 0.139392 0.139392 0.207566 0.207566 0.207566 0.268919 0.268919 0.268919 0.350184 0.350184 0.350184 0.43584 0.43584 0.43584 0.516391 0.516391 0.516391 0.588313 0.588313 0.588313 0.650587 0.650587 0.650587 0.720225 0.720225 0.720225 0.816454 0.816454 0.816454 1 1 1 1 1 1
  spline S22 degree 5 poles (5.4946, 315.7865) (5.458, 315.7865) (5.4214, 315.7832) (5.3851, 315.7752) (5.3116, 315.7464) (5.248, 315.6995) (5.217, 315.6713) (5.1474, 315.5982) (5.0885, 315.5162) (5.0565, 315.4666) (4.9905, 315.3543) (4.9325, 315.2378) (4.9026, 315.1733) (4.8431, 315.0378) (4.7885, 314.9002) (4.7611, 314.8284) (4.7074, 314.6821) (4.6568, 314.5347) (4.6319, 314.4598) (4.5834, 314.3087) (4.5375, 314.1568) (4.5152, 314.0803) (4.4717, 313.9271) (4.4307, 313.7732) (4.4108, 313.6961) (4.3727, 313.5434) (4.3371, 313.39) (4.3201, 313.314) (4.2882, 313.165) (4.2591, 313.0155) (4.2456, 312.9423) (4.2212, 312.8014) (4.2004, 312.66) (4.1913, 312.592) (4.1763, 312.4637) (4.1657, 312.335) (4.1619, 312.2746) (4.1572, 312.1629) (4.1579, 312.0511) (4.1595, 311.9999) (4.1651, 311.9075) (4.1765, 311.8156) (4.1829, 311.7748) (4.1971, 311.7027) (4.217, 311.6321) (4.227, 311.6016) (4.2473, 311.5482) (4.2726, 311.4972) (4.2848, 311.4753) (4.3089, 311.437) (4.3369, 311.4014) (4.3503, 311.3861) (4.3764, 311.3594) (4.4052, 311.3357) (4.4189, 311.3256) (4.445, 311.3085) (4.4728, 311.2945) (4.4858, 311.2889) (4.5098, 311.2802) (4.5346, 311.2744) (4.5457, 311.2725) (4.566, 311.2704) (4.5863, 311.2711) (4.5954, 311.272) (4.6141, 311.2754) (4.632, 311.2818) (4.6411, 311.2859) (4.6642, 311.2982) (4.6853, 311.3138) (4.6978, 311.3243) (4.729, 311.3537) (4.7566, 311.3865) (4.7727, 311.4077) (4.81, 311.4612) (4.8427, 311.5176) (4.8609, 311.5516) (4.9005, 311.6316) (4.9355, 311.7138) (4.9543, 311.7609) (4.994, 311.8667) (5.0298, 311.9739) (5.0486, 312.0332) (5.088, 312.1628) (5.1245, 312.2932) (5.1436, 312.3638) (5.1835, 312.5158) (5.2217, 312.6683) (5.2417, 312.7498) (5.2839, 312.9237) (5.3253, 313.0978) (5.3473, 313.1902) (5.3938, 313.3864) (5.4408, 313.5825) (5.4658, 313.6861) (5.5189, 313.9037) (5.5734, 314.1209) (5.6022, 314.2347) (5.66, 314.4628) (5.7152, 314.6918) (5.7418, 314.8066) (5.7862, 315.0171) (5.8184, 315.2289) (5.8287, 315.3258) (5.8378, 315.4643) (5.8208, 315.6049) (5.8116, 315.6435) (5.7838, 315.7544) (5.6589, 315.7736) (5.6193, 315.7822) (5.5475, 315.7875) (5.4946, 315.7865) knots 0 0 0 0 0 0 0.018098 0.018098 0.018098 0.038727 0.038727 0.038727 0.067909 0.067909 0.067909 0.103068 0.103068 0.103068 0.141102 0.141102 0.141102 0.180142 0.180142 0.180142 0.219574 0.219574 0.219574 0.258913 0.258913 0.258913 0.297449 0.297449 0.297449 0.334249 0.334249 0.334249 0.368164 0.368164 0.368164 0.398111 0.398111 0.398111 0.423438 0.423438 0.423438 0.44388 0.44388 0.44388 0.459721 0.459721 0.459721 0.472056 0.472056 0.472056 0.482091 0.482091 0.482091 0.490489 0.490489 0.490489 0.49748 0.49748 0.49748 0.503063 0.503063 0.503063 0.507534 0.507534 0.507534 0.512439 0.512439 0.512439 0.520472 0.520472 0.520472 0.533622 0.533622 0.533622 0.552686 0.552686 0.552686 0.577773 0.577773 0.577773 0.608556 0.608556 0.608556 0.644747 0.644747 0.644747 0.686282 0.686282 0.686282 0.733255 0.733255 0.733255 0.786008 0.786008 0.786008 0.844028 0.844028 0.844028 0.902436 0.902436 0.902436 0.950191 0.950191 0.950191 0.971416 0.971416 0.971416 1 1 1 1 1 1
  spline S23 degree 5 poles (7.2711, 316.433) (7.1348, 316.3126) (7.0252, 316.1584) (6.9653, 315.9781) (6.9228, 315.6502) (6.9473, 315.3204) (6.9644, 315.1749) (6.9943, 314.9179) (7.0043, 314.6596) (7.0009, 314.5477) (6.9763, 314.3138) (6.9416, 314.0814) (6.9273, 313.9584) (6.9156, 313.7025) (6.9299, 313.4467) (6.942, 313.3151) (6.9625, 313.0449) (6.9612, 312.7741) (6.9511, 312.6353) (6.91, 312.3444) (6.8459, 312.0568) (6.8086, 311.9068) (6.7375, 311.573) (6.7359, 311.2341) (6.7867, 311.0406) (7.0156, 310.7537) (7.3535, 310.6365) (7.5183, 310.6155) (7.8247, 310.5969) (8.1337, 310.6046) (8.2773, 310.6086) (8.5445, 310.6137) (8.8112, 310.6107) (8.9341, 310.6073) (9.1824, 310.5989) (9.431, 310.6027) (9.5568, 310.6111) (9.8242, 310.6536) (10.0745, 310.7578) (10.1988, 310.8348) (10.4185, 311.0279) (10.5746, 311.2754) (10.637, 311.4088) (10.7373, 311.679) (10.8045, 311.9594) (10.8324, 312.0981) (10.8797, 312.3651) (10.9182, 312.6333) (10.9352, 312.7617) (10.9649, 313.0045) (10.9898, 313.2479) (11.0005, 313.3627) (11.0185, 313.5786) (11.0358, 313.7946) (11.0441, 313.8957) (11.0631, 314.0944) (11.0904, 314.2921) (11.1068, 314.3888) (11.15, 314.6022) (11.2049, 314.813) (11.2369, 314.9282) (11.3093, 315.1847) (11.3707, 315.444) (11.3984, 315.5885) (11.425, 315.9116) (11.3411, 316.227) (11.2431, 316.3858) (10.9917, 316.5995) (10.682, 316.7031) (10.5358, 316.7325) (10.2691, 316.7737) (10, 316.801) (9.8791, 316.8131) (9.6638, 316.8345) (9.4482, 316.8486) (9.3535, 316.8521) (9.1777, 316.846) (9.0036, 316.8226) (8.9233, 316.8121) (8.7073, 316.7935) (8.4907, 316.7836) (8.3553, 316.7762) (8.043, 316.7507) (7.7358, 316.6888) (7.5648, 316.6362) (7.4038, 316.5504) (7.2711, 316.433) knots 0 0 0 0 0 0 0.047893 0.047893 0.047893 0.086516 0.086516 0.086516 0.115824 0.115824 0.115824 0.148309 0.148309 0.148309 0.183083 0.183083 0.183083 0.219473 0.219473 0.219473 0.260356 0.260356 0.260356 0.308516 0.308516 0.308516 0.351566 0.351566 0.351566 0.389474 0.389474 0.389474 0.421743 0.421743 0.421743 0.454809 0.454809 0.454809 0.492465 0.492465 0.492465 0.53091 0.53091 0.53091 0.568123 0.568123 0.568123 0.602156 0.602156 0.602156 0.632449 0.632449 0.632449 0.659122 0.659122 0.659122 0.684904 0.684904 0.684904 0.716349 0.716349 0.716349 0.754956 0.754956 0.754956 0.800583 0.800583 0.800583 0.839618 0.839618 0.839618 0.871602 0.871602 0.871602 0.896456 0.896456 0.896456 0.917756 0.917756 0.917756 0.953435 0.953435 0.953435 1 1 1 1 1 1
  spline S24 degree 5 poles (7.3778, 304.135) (7.1304, 304.1888) (6.8794, 304.2246) (6.6252, 304.2414) (6.1123, 304.2225) (5.6132, 304.1015) (5.3692, 304.0149) (4.895, 303.8111) (4.442, 303.563) (4.219, 303.4332) (3.8001, 303.1769) (3.4096, 302.8794) (3.2359, 302.7231) (2.886, 302.3416) (2.6005, 301.9095) (2.4589, 301.6628) (2.1896, 301.1351) (1.9758, 300.5823) (1.8796, 300.2893) (1.7057, 299.6303) (1.6042, 298.9565) (1.565, 298.5854) (1.5007, 297.7252) (1.5006, 296.8612) (1.5222, 296.3721) (1.6251, 295.4119) (1.9127, 294.4935) (2.1101, 294.0572) (2.7104, 293.2636) (3.6168, 292.8439) (4.116, 292.7468) (5.1851, 292.6835) (6.2413, 292.8973) (6.7854, 293.0672) (7.7258, 293.4708) (8.5523, 294.0651) (8.8886, 294.3656) (9.4005, 294.976) (9.7521, 295.6875) (9.8729, 296.0108) (10.0652, 296.6358) (10.2097, 297.2738) (10.2716, 297.5777) (10.3726, 298.1976) (10.4039, 298.825) (10.3965, 299.1432) (10.3362, 299.8096) (10.2063, 300.4662) (10.1239, 300.8079) (9.9568, 301.4333) (9.7519, 302.0475) (9.6507, 302.3253) (9.4388, 302.8132) (9.124, 303.2412) (8.9573, 303.4084) (8.5657, 303.7071) (8.1197, 303.9172) (7.8771, 304.0066) (7.6296, 304.0803) (7.3778, 304.135) knots 0 0 0 0 0 0 0.03868 0.03868 0.03868 0.078046 0.078046 0.078046 0.117494 0.117494 0.117494 0.152981 0.152981 0.152981 0.196364 0.196364 0.196364 0.243409 0.243409 0.243409 0.300349 0.300349 0.300349 0.375222 0.375222 0.375222 0.446982 0.446982 0.446982 0.522898 0.522898 0.522898 0.609801 0.609801 0.609801 0.677903 0.677903 0.677903 0.730401 0.730401 0.730401 0.777785 0.777785 0.777785 0.826232 0.826232 0.826232 0.879911 0.879911 0.879911 0.925119 0.925119 0.925119 0.960628 0.960628 0.960628 1 1 1 1 1 1
  spline S25 degree 5 poles (-3.492, 311.6401) (-3.4432, 311.9073) (-3.4074, 312.1777) (-3.3799, 312.4458) (-3.3258, 312.9119) (-3.1198, 313.3343) (-2.9917, 313.4839) (-2.709, 313.7409) (-2.3843, 313.9472) (-2.2159, 314.0347) (-1.9072, 314.1747) (-1.5669, 314.1693) (-1.4284, 314.1185) (-1.1187, 313.9419) (-0.8961, 313.6522) (-0.7995, 313.4612) (-0.608, 312.9829) (-0.4599, 312.4907) (-0.3532, 312.2075) (-0.0823, 311.6218) (0.2256, 311.0526) (0.3615, 310.7392) (0.5514, 310.4386) (0.8029, 310.203) knots 0 0 0 0 0 0 0.164362 0.164362 0.164362 0.280025 0.280025 0.280025 0.395497 0.395497 0.395497 0.480465 0.480465 0.480465 0.609393 0.609393 0.609393 0.791563 0.791563 0.791563 1 1 1 1 1 1
  spline S26 degree 5 poles (0.803, 310.2028) (0.4151, 309.8834) (0.0326, 309.5567) (-0.347, 309.2303) (-1.0035, 308.758) (-1.7531, 308.4726) (-2.0416, 308.3957) (-2.5567, 308.338) (-3.0653, 308.4165) (-3.2754, 308.4741) (-3.6663, 308.6224) (-4.0268, 308.8344) (-4.1913, 308.9514) (-4.5084, 309.2227) (-4.7963, 309.5246) (-4.9416, 309.6838) (-5.0971, 309.8351) (-5.2661, 309.9694) knots 0 0 0 0 0 0 0.351173 0.351173 0.351173 0.557889 0.557889 0.557889 0.708807 0.708807 0.708807 0.849112 0.849112 0.849112 1 1 1 1 1 1
  spline S27 degree 5 poles (-7.1927, 309.2254) (-7.328, 309.2045) (-7.4633, 309.184) (-7.5985, 309.162) (-7.8733, 309.1129) (-8.146, 309.0526) (-8.2841, 309.0183) (-8.5738, 308.9379) (-8.8597, 308.8446) (-9.0093, 308.7926) (-9.3349, 308.6741) (-9.6569, 308.546) (-9.8308, 308.4741) (-10.203, 308.3143) (-10.5707, 308.1444) (-10.7663, 308.0507) (-11.1643, 307.8542) (-11.5575, 307.6482) (-11.7573, 307.5406) (-12.136, 307.3311) (-12.5097, 307.1129) (-12.6862, 307.007) (-13.0039, 306.8109) (-13.3167, 306.6069) (-13.4558, 306.5139) (-13.6783, 306.3623) (-13.8925, 306.1997) (-13.9708, 306.135) (-14.0805, 306.0411) (-14.1605, 305.9198) (-14.1697, 305.8766) (-14.1839, 305.7024) (-14.1479, 305.5281) (-14.1178, 305.4002) (-14.0198, 305.0648) (-13.8998, 304.7375) (-13.8222, 304.5354) (-13.6531, 304.1082) (-13.4775, 303.6833) (-13.3838, 303.4588) (-13.1906, 303.004) (-12.9895, 302.5527) (-12.8851, 302.3246) (-12.6721, 301.8732) (-12.4478, 301.4272) (-12.3333, 301.2068) (-12.1054, 300.7842) (-11.8656, 300.3682) (-11.7474, 300.1688) (-11.5151, 299.7852) (-11.284, 299.4009) (-11.1744, 299.214) (-11.0425, 298.9726) (-10.9239, 298.7248) (-10.8995, 298.6721) (-10.8758, 298.619) (-10.8528, 298.5656) knots 0 0 0 0 0 0 0.042998 0.042998 0.042998 0.087674 0.087674 0.087674 0.137414 0.137414 0.137414 0.196496 0.196496 0.196496 0.264622 0.264622 0.264622 0.335889 0.335889 0.335889 0.400534 0.400534 0.400534 0.45314 0.45314 0.45314 0.485005 0.485005 0.485005 0.498195 0.498195 0.498195 0.539795 0.539795 0.539795 0.60773 0.60773 0.60773 0.684143 0.684143 0.684143 0.762914 0.762914 0.762914 0.840903 0.840903 0.840903 0.913705 0.913705 0.913705 0.981752 0.981752 0.981752 1 1 1 1 1 1
  spline S28 degree 5 poles (-11.2057, 293.888) (-11.3012, 293.8342) (-11.3984, 293.7834) (-11.4969, 293.7352) (-11.786, 293.6005) (-12.082, 293.4811) (-12.2757, 293.4033) (-12.7014, 293.2584) (-13.1544, 293.257) (-13.3958, 293.3243) (-13.7771, 293.5624) (-14.0403, 293.9221) (-14.1375, 294.1018) (-14.3154, 294.4905) (-14.4197, 294.9056) (-14.4488, 295.1301) (-14.4137, 295.6636) (-14.1352, 296.1311) (-13.9135, 296.3454) (-13.3477, 296.7671) (-12.6785, 297.0115) (-12.2841, 297.1007) (-11.8826, 297.1407) (-11.4813, 297.1366) knots 0 0 0 0 0 0 0.065128 0.065128 0.065128 0.189501 0.189501 0.189501 0.32979 0.32979 0.32979 0.450518 0.450518 0.450518 0.582986 0.582986 0.582986 0.761663 0.761663 0.761663 1 1 1 1 1 1